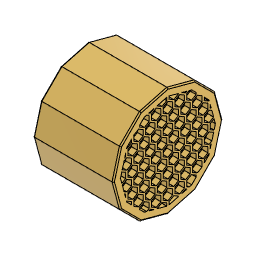
Speaker_End_Cap (Autodesk Fusion 360 design; units mm, degrees)
Autodesk Fusion 360 part; units mm, degrees
note: some values were not read from the file. Set by a fixed rule: which sketch regions a step uses.
sketch "Sketch1" plane through (0, 0, 0) normal (1, 0, 0) x (0, 1, 0)
  line L0 (22, 0) -> (19.0526, 11)
  line L1 (19.0526, 11) -> (11, 19.0526)
  line L2 (11, 19.0526) -> (0, 22)
  line L3 (0, 22) -> (-11, 19.0526)
  line L4 (-11, 19.0526) -> (-19.0526, 11)
  line L5 (-19.0526, 11) -> (-22, 0)
  line L6 (-22, 0) -> (-19.0526, -11)
  line L7 (-19.0526, -11) -> (-11, -19.0526)
  line L8 (-11, -19.0526) -> (0, -22)
  line L9 (0, -22) -> (11, -19.0526)
  line L10 (11, -19.0526) -> (19.0526, -11)
  line L11 (19.0526, -11) -> (22, 0)
  line L12 (20.1733, 11.647) -> (11.647, 20.1733)
  line L13 (11.647, 20.1733) -> (0, 23.2941)
  line L14 (0, 23.2941) -> (-11.647, 20.1733)
  line L15 (-11.647, 20.1733) -> (-20.1733, 11.647)
  line L16 (-20.1733, 11.647) -> (-23.2941, 0)
  line L17 (-23.2941, 0) -> (-20.1733, -11.647)
  line L18 (-20.1733, -11.647) -> (-11.647, -20.1733)
  line L19 (-11.647, -20.1733) -> (0, -23.2941)
  line L20 (0, -23.2941) -> (11.647, -20.1733)
  line L21 (11.647, -20.1733) -> (20.1733, -11.647)
  line L22 (20.1733, -11.647) -> (23.2941, 0)
  line L23 (23.2941, 0) -> (20.1733, 11.647)
  dimension "d1" = 22
  dimension "d2" = 1.25
  measures "d1" distance of L0.start origin
extrude "Extrude1" add sketch "Sketch1" along normal blind 2.5 contours L0 L1 L2 L3 L4 L5 L6 L7 L8 L9 L10 L11 | L12 L13 L14 L15 L16 L17 L18 L19 L20 L21 L22 L23
extrude "Extrude3" add sketch "Sketch1" against normal blind 31.5
fillet "Rounded Edges" radius 0.5 12 edges at (2.5, -5.8235, 21.7337) (2.5, 5.8235, 21.7337) (2.5, 15.9102, 15.9102) (2.5, 21.7337, 5.8235) (2.5, 21.7337, -5.8235) (2.5, 15.9102, -15.9102) (2.5, 5.8235, -21.7337) (2.5, -5.8235, -21.7337) (2.5, -15.9102, -15.9102) (2.5, -21.7337, -5.8235) (2.5, -21.7337, 5.8235) (2.5, -15.9102, 15.9102)
fillet "Rounded Edges" radius 0.5 12 edges at (-31.5, -15.9102, 15.9102) (-31.5, -5.8235, 21.7337) (-31.5, 5.8235, 21.7337) (-31.5, 15.9102, 15.9102) (-31.5, 21.7337, 5.8235) (-31.5, 21.7337, -5.8235) (-31.5, 15.9102, -15.9102) (-31.5, 5.8235, -21.7337) (-31.5, -5.8235, -21.7337) (-31.5, -15.9102, -15.9102) (-31.5, -21.7337, -5.8235) (-31.5, -21.7337, 5.8235)
sketch "Speaker Grill" plane through (2.5, 0, 0) normal (1, 0, 0) x (0, 1, 0)
  line L0 (0, -22.7765) -> (11.3882, -19.725)
  line L1 (11.3882, -19.725) -> (19.725, -11.3882)
  line L2 (19.725, -11.3882) -> (22.7765, 0)
  line L3 (22.7765, 0) -> (19.725, 11.3882)
  line L4 (19.725, 11.3882) -> (11.3882, 19.725)
  line L5 (11.3882, 19.725) -> (0, 22.7765)
  line L6 (0, 22.7765) -> (-11.3882, 19.725)
  line L7 (-11.3882, 19.725) -> (-19.725, 11.3882)
  line L8 (-19.725, 11.3882) -> (-22.7765, 0)
  line L9 (-22.7765, 0) -> (-19.725, -11.3882)
  line L10 (-19.725, -11.3882) -> (-11.3882, -19.725)
  line L11 (-11.3882, -19.725) -> (0, -22.7765)
  line L12 (-17.4836, 10.0941) -> (-20.1883, 0)
  line L13 (-20.1883, 0) -> (-17.4836, -10.0941)
  line L14 (-17.4836, -10.0941) -> (-10.0941, -17.4836)
  line L15 (-10.0941, -17.4836) -> (0, -20.1883)
  line L16 (0, -20.1883) -> (10.0941, -17.4836)
  line L17 (10.0941, -17.4836) -> (17.4836, -10.0941)
  line L18 (17.4836, -10.0941) -> (20.1883, 0)
  line L19 (20.1883, 0) -> (17.4836, 10.0941)
  line L20 (17.4836, 10.0941) -> (10.0941, 17.4836)
  line L21 (10.0941, 17.4836) -> (0, 20.1883)
  line L22 (0, 20.1883) -> (-10.0941, 17.4836)
  line L23 (-10.0941, 17.4836) -> (-17.4836, 10.0941)
  line L24 (2, 1.1547) -> (0, 2.3094)
  line L25 (0, 2.3094) -> (-2, 1.1547)
  line L26 (-2, 1.1547) -> (-2, -1.1547)
  line L27 (-2, -1.1547) -> (0, -2.3094)
  line L28 (0, -2.3094) -> (2, -1.1547)
  line L29 (2, -1.1547) -> (2, 1.1547)
  line L30 (7, 1.1547) -> (5, 2.3094)
  line L31 (5, 2.3094) -> (3, 1.1547)
  line L32 (3, 1.1547) -> (3, -1.1547)
  line L33 (3, -1.1547) -> (5, -2.3094)
  line L34 (5, -2.3094) -> (7, -1.1547)
  line L35 (7, -1.1547) -> (7, 1.1547)
  line L36 (12, 1.1547) -> (10, 2.3094)
  line L37 (10, 2.3094) -> (8, 1.1547)
  line L38 (8, 1.1547) -> (8, -1.1547)
  line L39 (8, -1.1547) -> (10, -2.3094)
  line L40 (10, -2.3094) -> (12, -1.1547)
  line L41 (12, -1.1547) -> (12, 1.1547)
  line L42 (17, 1.1547) -> (15, 2.3094)
  line L43 (15, 2.3094) -> (13, 1.1547)
  line L44 (13, 1.1547) -> (13, -1.1547)
  line L45 (13, -1.1547) -> (15, -2.3094)
  line L46 (15, -2.3094) -> (17, -1.1547)
  line L47 (17, -1.1547) -> (17, 1.1547)
  line L48 (-7, -1.1547) -> (-5, -2.3094)
  line L49 (-5, -2.3094) -> (-3, -1.1547)
  line L50 (-3, -1.1547) -> (-3, 1.1547)
  line L51 (-3, 1.1547) -> (-5, 2.3094)
  line L52 (-5, 2.3094) -> (-7, 1.1547)
  line L53 (-7, 1.1547) -> (-7, -1.1547)
  line L54 (-12, -1.1547) -> (-10, -2.3094)
  line L55 (-10, -2.3094) -> (-8, -1.1547)
  line L56 (-8, -1.1547) -> (-8, 1.1547)
  line L57 (-8, 1.1547) -> (-10, 2.3094)
  line L58 (-10, 2.3094) -> (-12, 1.1547)
  line L59 (-12, 1.1547) -> (-12, -1.1547)
  line L60 (-17, -1.1547) -> (-15, -2.3094)
  line L61 (-15, -2.3094) -> (-13, -1.1547)
  line L62 (-13, -1.1547) -> (-13, 1.1547)
  line L63 (-13, 1.1547) -> (-15, 2.3094)
  line L64 (-15, 2.3094) -> (-17, 1.1547)
  line L65 (-17, 1.1547) -> (-17, -1.1547)
  line L66 (-18, 1.1547) -> (-20, 2.3094)
  line L67 (-20, 2.3094) -> (-22, 1.1547)
  line L68 (-22, 1.1547) -> (-22, -1.1547)
  line L69 (-22, -1.1547) -> (-20, -2.3094)
  line L70 (-20, -2.3094) -> (-18, -1.1547)
  line L71 (-18, -1.1547) -> (-18, 1.1547)
  line L72 (18, -1.1547) -> (20, -2.3094)
  line L73 (20, -2.3094) -> (22, -1.1547)
  line L74 (22, -1.1547) -> (22, 1.1547)
  line L75 (22, 1.1547) -> (20, 2.3094)
  line L76 (20, 2.3094) -> (18, 1.1547)
  line L77 (18, 1.1547) -> (18, -1.1547)
  line L78 (2.493, -1.6981) -> (0.4965, -2.8589)
  line L79 (0.4965, -2.8589) -> (0.5035, -5.1683)
  line L80 (0.5035, -5.1683) -> (2.507, -6.3169)
  line L81 (2.507, -6.3169) -> (4.5035, -5.1561)
  line L82 (4.5035, -5.1561) -> (4.4965, -2.8467)
  line L83 (4.4965, -2.8467) -> (2.493, -1.6981)
  line L84 (9.5035, -5.1561) -> (9.4965, -2.8467)
  line L85 (7.507, -6.3169) -> (9.5035, -5.1561)
  line L86 (5.5035, -5.1683) -> (7.507, -6.3169)
  line L87 (5.4965, -2.8589) -> (5.5035, -5.1683)
  line L88 (7.493, -1.6981) -> (5.4965, -2.8589)
  line L89 (9.4965, -2.8467) -> (7.493, -1.6981)
  line L90 (10.4965, -2.8589) -> (10.5035, -5.1683)
  line L91 (14.4965, -2.8467) -> (12.493, -1.6981)
  line L92 (12.507, -6.3169) -> (14.5035, -5.1561)
  line L93 (10.5035, -5.1683) -> (12.507, -6.3169)
  line L94 (12.493, -1.6981) -> (10.4965, -2.8589)
  line L95 (14.5035, -5.1561) -> (14.4965, -2.8467)
  line L96 (9.5, 2.8453) -> (9.5, 5.1547)
  line L97 (-4.5, 5.1547) -> (-4.5, 2.8453)
  line L98 (-2.5, 6.3094) -> (-4.5, 5.1547)
  line L99 (-2.5, 1.6906) -> (-0.5, 2.8453)
  line L100 (-5.5, 5.1547) -> (-7.5, 6.3094)
  line L101 (-9.5, 2.8453) -> (-7.5, 1.6906)
  line L102 (-7.5, 6.3094) -> (-9.5, 5.1547)
  line L103 (-7.5, 1.6906) -> (-5.5, 2.8453)
  line L104 (-4.5, 2.8453) -> (-2.5, 1.6906)
  line L105 (-0.5, 2.8453) -> (-0.5, 5.1547)
  line L106 (5.5, 5.1547) -> (5.5, 2.8453)
  line L107 (4.5, 2.8453) -> (4.5, 5.1547)
  line L108 (-9.5, 5.1547) -> (-9.5, 2.8453)
  line L109 (-5.5, 2.8453) -> (-5.5, 5.1547)
  line L110 (0.5, 5.1547) -> (0.5, 2.8453)
  line L111 (9.5, 5.1547) -> (7.5, 6.3094)
  line L112 (2.5, 1.6906) -> (4.5, 2.8453)
  line L113 (5.5, 2.8453) -> (7.5, 1.6906)
  line L114 (0.5, 2.8453) -> (2.5, 1.6906)
  line L115 (4.5, 5.1547) -> (2.5, 6.3094)
  line L116 (7.5, 6.3094) -> (5.5, 5.1547)
  line L117 (2.5, 6.3094) -> (0.5, 5.1547)
  line L118 (7.5, 1.6906) -> (9.5, 2.8453)
  line L119 (-0.5, 5.1547) -> (-2.5, 6.3094)
  line L120 (10.5, 2.8453) -> (12.5, 1.6906)
  line L121 (10.5, 5.1547) -> (10.5, 2.8453)
  line L122 (12.5, 6.3094) -> (10.5, 5.1547)
  line L123 (14.5, 5.1547) -> (12.5, 6.3094)
  line L124 (14.5, 2.8453) -> (14.5, 5.1547)
  line L125 (12.5, 1.6906) -> (14.5, 2.8453)
  line L126 (-10.5, 5.1547) -> (-12.5, 6.3094)
  line L127 (-12.5, 6.3094) -> (-14.5, 5.1547)
  line L128 (-14.5, 5.1547) -> (-14.5, 2.8453)
  line L129 (-14.5, 2.8453) -> (-12.5, 1.6906)
  line L130 (-12.5, 1.6906) -> (-10.5, 2.8453)
  line L131 (-10.5, 2.8453) -> (-10.5, 5.1547)
  line L132 (-15.5, 5.1547) -> (-17.5, 6.3094)
  line L133 (-17.5, 6.3094) -> (-19.5, 5.1547)
  line L134 (-19.5, 5.1547) -> (-19.5, 2.8453)
  line L135 (-19.5, 2.8453) -> (-17.5, 1.6906)
  line L136 (-17.5, 1.6906) -> (-15.5, 2.8453)
  line L137 (-15.5, 2.8453) -> (-15.5, 5.1547)
  line L138 (19.5, 2.8453) -> (19.5, 5.1547)
  line L139 (19.5, 5.1547) -> (17.5, 6.3094)
  line L140 (17.5, 6.3094) -> (15.5, 5.1547)
  line L141 (15.5, 5.1547) -> (15.5, 2.8453)
  line L142 (15.5, 2.8453) -> (17.5, 1.6906)
  line L143 (17.5, 1.6906) -> (19.5, 2.8453)
  line L144 (19.5035, -5.1561) -> (19.4965, -2.8467)
  line L145 (19.4965, -2.8467) -> (17.493, -1.6981)
  line L146 (17.493, -1.6981) -> (15.4965, -2.8589)
  line L147 (15.4965, -2.8589) -> (15.5035, -5.1683)
  line L148 (15.5035, -5.1683) -> (17.507, -6.3169)
  line L149 (17.507, -6.3169) -> (19.5035, -5.1561)
  line L150 (-15.4965, -5.1561) -> (-15.5035, -2.8467)
  line L151 (-15.5035, -2.8467) -> (-17.507, -1.6981)
  line L152 (-17.507, -1.6981) -> (-19.5035, -2.8589)
  line L153 (-19.5035, -2.8589) -> (-19.4965, -5.1683)
  line L154 (-19.4965, -5.1683) -> (-17.493, -6.3169)
  line L155 (-17.493, -6.3169) -> (-15.4965, -5.1561)
  line L156 (-14.5035, -2.8589) -> (-14.4965, -5.1683)
  line L157 (-12.507, -1.6981) -> (-14.5035, -2.8589)
  line L158 (-10.5035, -2.8467) -> (-12.507, -1.6981)
  line L159 (-10.4965, -5.1561) -> (-10.5035, -2.8467)
  line L160 (-12.493, -6.3169) -> (-10.4965, -5.1561)
  line L161 (-14.4965, -5.1683) -> (-12.493, -6.3169)
  line L162 (-9.4965, -5.1683) -> (-7.493, -6.3169)
  line L163 (-9.5035, -2.8589) -> (-9.4965, -5.1683)
  line L164 (-7.507, -1.6981) -> (-9.5035, -2.8589)
  line L165 (-5.5035, -2.8467) -> (-7.507, -1.6981)
  line L166 (-5.4965, -5.1561) -> (-5.5038, -2.7646)
  line L167 (-7.493, -6.3169) -> (-5.4965, -5.1561)
  line L168 (-4.5035, -2.8589) -> (-4.4965, -5.1683)
  line L169 (-2.507, -1.6981) -> (-4.5035, -2.8589)
  line L170 (-0.5035, -2.8467) -> (-2.507, -1.6981)
  line L171 (-0.4965, -5.1561) -> (-0.5035, -2.8467)
  line L172 (-2.493, -6.3169) -> (-0.4965, -5.1561)
  line L173 (-4.4965, -5.1683) -> (-2.493, -6.3169)
  line L174 (-4.5, 13.1547) -> (-4.5, 10.8453)
  line L175 (-2.5, 14.3094) -> (-4.5, 13.1547)
  line L176 (9.5, 10.8453) -> (9.5, 13.1547)
  line L177 (10.5, 13.1547) -> (10.5, 10.8453)
  line L178 (-2.5, 9.6906) -> (-0.5, 10.8453)
  line L179 (-15.5, 10.8453) -> (-15.5, 13.1547)
  line L180 (-5.007, 10.3019) -> (-7.0035, 9.1411)
  line L181 (2.5, 9.6906) -> (4.5, 10.8453)
  line L182 (-3.0035, 9.1533) -> (-5.007, 10.3019)
  line L183 (8, 14.8453) -> (10, 13.6906)
  line L184 (-6.9965, 6.8317) -> (-4.993, 5.6831)
  line L185 (3, 14.8453) -> (5, 13.6906)
  line L186 (-12.5, 14.3094) -> (-14.5, 13.1547)
  line L187 (-2, 17.1547) -> (-2, 14.8453)
  line L188 (2, 17.1547) -> (0, 18.3094)
  line L189 (7.5, 9.6906) -> (9.5, 10.8453)
  line L190 (-0.007, 10.3019) -> (-2.0035, 9.1411)
  line L191 (-8.0035, 9.1533) -> (-10.007, 10.3019)
  line L192 (-7.0035, 9.1411) -> (-6.9965, 6.8317)
  line L193 (-14.5, 10.8453) -> (-12.5, 9.6906)
  line L194 (-7, 17.1547) -> (-7, 14.8453)
  line L195 (0.007, 5.6831) -> (2.0035, 6.8439)
  line L196 (0.5, 10.8453) -> (2.5, 9.6906)
  line L197 (4.5, 13.1547) -> (2.5, 14.3094)
  line L198 (7.5, 14.3094) -> (5.5, 13.1547)
  line L199 (-14.993, 5.6831) -> (-12.9965, 6.8439)
  line L200 (7, 17.1547) -> (5, 18.3094)
  line L201 (2, 14.8453) -> (2, 17.1547)
  line L202 (-12.5, 9.6906) -> (-10.5, 10.8453)
  line L203 (-17.0035, 9.1411) -> (-16.9965, 6.8317)
  line L204 (-12.9965, 6.8439) -> (-13.0035, 9.1533)
  line L205 (0, 13.6906) -> (2, 14.8453)
  line L206 (6.9965, 9.1533) -> (4.993, 10.3019)
  line L207 (-1.9965, 6.8317) -> (0.007, 5.6831)
  line L208 (4.993, 10.3019) -> (2.9965, 9.1411)
  line L209 (-10, 13.6906) -> (-8, 14.8453)
  line L210 (-10, 18.3094) -> (-12, 17.1547)
  line L211 (8.0035, 6.8317) -> (10.007, 5.6831)
  line L212 (5, 13.6906) -> (7, 14.8453)
  line L213 (-7.5, 9.6906) -> (-5.5, 10.8453)
  line L214 (-10.5, 13.1547) -> (-12.5, 14.3094)
  line L215 (-7.9965, 6.8439) -> (-8.0035, 9.1533)
  line L216 (-16.9965, 6.8317) -> (-14.993, 5.6831)
  line L217 (5.007, 5.6831) -> (7.0035, 6.8439)
  line L218 (5, 18.3094) -> (3, 17.1547)
  line L219 (-5, 13.6906) -> (-3, 14.8453)
  line L220 (-12.0035, 9.1411) -> (-11.9965, 6.8317)
  line L221 (-3, 17.1547) -> (-5, 18.3094)
  line L222 (-12, 17.1547) -> (-12, 14.8453)
  line L223 (-9.993, 5.6831) -> (-7.9965, 6.8439)
  line L224 (7, 14.8453) -> (7, 17.1547)
  line L225 (-5.5, 13.1547) -> (-7.5, 14.3094)
  line L226 (-3, 14.8453) -> (-3, 17.1547)
  line L227 (10, 18.3094) -> (8, 17.1547)
  line L228 (-15.007, 10.3019) -> (-17.0035, 9.1411)
  line L229 (-2.9965, 6.8439) -> (-3.0035, 9.1533)
  line L230 (7.0035, 6.8439) -> (6.9965, 9.1533)
  line L231 (1.9965, 9.1533) -> (-0.007, 10.3019)
  line L232 (9.993, 10.3019) -> (7.9965, 9.1411)
  line L233 (-11.9965, 6.8317) -> (-9.993, 5.6831)
  line L234 (-13.0035, 9.1533) -> (-15.007, 10.3019)
  line L235 (5.5, 10.8453) -> (7.5, 9.6906)
  line L236 (-4.993, 5.6831) -> (-2.9965, 6.8439)
  line L237 (-5, 18.3094) -> (-7, 17.1547)
  line L238 (-10.007, 10.3019) -> (-12.0035, 9.1411)
  line L239 (9.5, 13.1547) -> (7.5, 14.3094)
  line L240 (5.5, 13.1547) -> (5.5, 10.8453)
  line L241 (-7, 14.8453) -> (-5, 13.6906)
  line L242 (-2, 14.8453) -> (0, 13.6906)
  line L243 (4.5, 10.8453) -> (4.5, 13.1547)
  line L244 (-0.5, 10.8453) -> (-0.5, 13.1547)
  line L245 (0.5, 13.1547) -> (0.5, 10.8453)
  line L246 (-14.5, 13.1547) -> (-14.5, 10.8453)
  line L247 (-9.5, 13.1547) -> (-9.5, 10.8453)
  line L248 (-10.5, 10.8453) -> (-10.5, 13.1547)
  line L249 (-5.5, 10.8453) -> (-5.5, 13.1547)
  line L250 (-8, 14.8453) -> (-8, 17.1547)
  line L251 (-15.5, 13.1547) -> (-17.5, 14.3094)
  line L252 (-8, 17.1547) -> (-10, 18.3094)
  line L253 (-7.5, 14.3094) -> (-9.5, 13.1547)
  line L254 (-9.5, 10.8453) -> (-7.5, 9.6906)
  line L255 (2.5, 14.3094) -> (0.5, 13.1547)
  line L256 (3.0035, 6.8317) -> (5.007, 5.6831)
  line L257 (2.9965, 9.1411) -> (3.0035, 6.8317)
  line L258 (0, 18.3094) -> (-2, 17.1547)
  line L259 (-4.5, 10.8453) -> (-2.5, 9.6906)
  line L260 (-17.5, 9.6906) -> (-15.5, 10.8453)
  line L261 (7.9965, 9.1411) -> (8.0035, 6.8317)
  line L262 (-2.0035, 9.1411) -> (-1.9965, 6.8317)
  line L263 (-0.5, 13.1547) -> (-2.5, 14.3094)
  line L264 (2.0035, 6.8439) -> (1.9965, 9.1533)
  line L265 (3, 17.1547) -> (3, 14.8453)
  line L266 (8, 17.1547) -> (8, 14.8453)
  line L267 (-12, 14.8453) -> (-10, 13.6906)
  line L268 (14.5, 10.8453) -> (14.5, 13.1547)
  line L269 (14.993, 10.3019) -> (12.9965, 9.1411)
  line L270 (19.5, 13.1547) -> (17.5, 14.3094)
  line L271 (12, 14.8453) -> (12, 17.1547)
  line L272 (16.9965, 9.1533) -> (14.993, 10.3019)
  line L273 (19.5, 10.8453) -> (19.5, 13.1547)
  line L274 (12.0035, 6.8439) -> (11.9965, 9.1533)
  line L275 (17.0035, 6.8439) -> (16.9965, 9.1533)
  line L276 (12.5, 9.6906) -> (14.5, 10.8453)
  line L277 (12.9965, 9.1411) -> (13.0035, 6.8317)
  line L278 (14.5, 13.1547) -> (12.5, 14.3094)
  line L279 (15.5, 10.8453) -> (17.5, 9.6906)
  line L280 (17.5, 14.3094) -> (15.5, 13.1547)
  line L281 (17.5, 9.6906) -> (19.5, 10.8453)
  line L282 (15.5, 13.1547) -> (15.5, 10.8453)
  line L283 (13.0035, 6.8317) -> (15.007, 5.6831)
  line L284 (15.007, 5.6831) -> (17.0035, 6.8439)
  line L285 (10.5, 10.8453) -> (12.5, 9.6906)
  line L286 (12.5, 14.3094) -> (10.5, 13.1547)
  line L287 (10, 13.6906) -> (12, 14.8453)
  line L288 (12, 17.1547) -> (10, 18.3094)
  line L289 (10.007, 5.6831) -> (12.0035, 6.8439)
  line L290 (11.9965, 9.1533) -> (9.993, 10.3019)
  line L291 (-17.9965, 6.8439) -> (-18.0035, 9.1533)
  line L292 (-18.0035, 9.1533) -> (-20.007, 10.3019)
  line L293 (-20.007, 10.3019) -> (-22.0035, 9.1411)
  line L294 (-22.0035, 9.1411) -> (-21.9965, 6.8317)
  line L295 (-21.9965, 6.8317) -> (-19.993, 5.6831)
  line L296 (-19.993, 5.6831) -> (-17.9965, 6.8439)
  line L297 (-19.5, 10.8453) -> (-17.5, 9.6906)
  line L298 (-19.5, 13.1547) -> (-19.5, 10.8453)
  line L299 (-17.5, 14.3094) -> (-19.5, 13.1547)
  line L300 (4.5, 21.1547) -> (2.5, 22.3094)
  line L301 (2.5, 22.3094) -> (0.5, 21.1547)
  line L302 (0.5, 21.1547) -> (0.5, 18.8453)
  line L303 (0.5, 18.8453) -> (2.5, 17.6906)
  line L304 (2.5, 17.6906) -> (4.5, 18.8453)
  line L305 (4.5, 18.8453) -> (4.5, 21.1547)
  line L306 (-0.5, 21.1547) -> (-2.5, 22.3094)
  line L307 (-2.5, 22.3094) -> (-4.5, 21.1547)
  line L308 (-4.5, 21.1547) -> (-4.5, 18.8453)
  line L309 (-4.5, 18.8453) -> (-2.5, 17.6906)
  line L310 (-2.5, 17.6906) -> (-0.5, 18.8453)
  line L311 (-0.5, 18.8453) -> (-0.5, 21.1547)
  line L312 (5.5, 21.1547) -> (5.5, 18.8453)
  line L313 (9.5, 21.1547) -> (7.5, 22.3094)
  line L314 (7.5, 22.3094) -> (5.5, 21.1547)
  line L315 (5.5, 18.8453) -> (7.5, 17.6906)
  line L316 (7.5, 17.6906) -> (9.5, 18.8453)
  line L317 (9.5, 18.8453) -> (9.5, 21.1547)
  line L318 (-5.5, 21.1547) -> (-7.5, 22.3094)
  line L319 (-7.5, 22.3094) -> (-9.5, 21.1547)
  line L320 (-9.5, 21.1547) -> (-9.5, 18.8453)
  line L321 (-9.5, 18.8453) -> (-7.5, 17.6906)
  line L322 (-7.5, 17.6906) -> (-5.5, 18.8453)
  line L323 (-5.5, 18.8453) -> (-5.5, 21.1547)
  line L324 (7.0035, -9.1561) -> (6.9965, -6.8467)
  line L325 (-5, -18.3094) -> (-3, -17.1547)
  line L326 (-19.5, -10.8453) -> (-19.5, -13.1547)
  line L327 (12.0035, -9.1561) -> (11.9965, -6.8467)
  line L328 (12, -17.1547) -> (12, -14.8453)
  line L329 (7, -17.1547) -> (7, -14.8453)
  line L330 (-4.4965, -21.1683) -> (-2.493, -22.3169)
  line L331 (-5, -13.6906) -> (-7, -14.8453)
  line L332 (12.9965, -6.8589) -> (13.0035, -9.1683)
  line L333 (7.507, -22.3169) -> (9.5035, -21.1561)
  line L334 (-9.5035, -18.8589) -> (-9.4965, -21.1683)
  line L335 (2, -17.1547) -> (2, -14.8453)
  line L336 (-7, -17.1547) -> (-5, -18.3094)
  line L337 (-12, -17.1547) -> (-10, -18.3094)
  line L338 (-5.5, -13.1547) -> (-5.5, -10.8453)
  line L339 (-9.5, -13.1547) -> (-7.5, -14.3094)
  line L340 (2.493, -17.6981) -> (0.4965, -18.8589)
  line L341 (3, -14.8453) -> (3, -17.1547)
  line L342 (-15.5, -13.1547) -> (-15.5, -10.8453)
  line L343 (2.0035, -9.1561) -> (1.9965, -6.8467)
  line L344 (-12.8895, -14.6882) -> (-12.8895, -14.6712)
  line L345 (-2.493, -22.3169) -> (-0.4965, -21.1561)
  line L346 (8, -14.8453) -> (8, -17.1547)
  line L347 (-9.5, -10.8453) -> (-9.5, -13.1547)
  line L348 (-4.5, -10.8453) -> (-4.5, -13.1547)
  line L349 (4.4965, -18.8467) -> (2.493, -17.6981)
  line L350 (-0.4965, -21.1561) -> (-0.5035, -18.8467)
  line L351 (-17.5, -14.3094) -> (-15.5, -13.1547)
  line L352 (-15.5, -10.8453) -> (-17.5, -9.6906)
  line L353 (10, -18.3094) -> (12, -17.1547)
  line L354 (9.5035, -21.1561) -> (9.4965, -18.8467)
  line L355 (7.493, -17.6981) -> (5.4965, -18.8589)
  line L356 (5.5035, -21.1683) -> (7.507, -22.3169)
  line L357 (5, -18.3094) -> (7, -17.1547)
  line L358 (0.4965, -18.8589) -> (0.5035, -21.1683)
  line L359 (8, -17.1547) -> (10, -18.3094)
  line L360 (2.507, -22.3169) -> (4.5035, -21.1561)
  line L361 (0, -18.3094) -> (2, -17.1547)
  line L362 (0, -13.6906) -> (-2, -14.8453)
  line L363 (5.4965, -18.8589) -> (5.5035, -21.1683)
  line L364 (1.9965, -6.8467) -> (-0.007, -5.6981)
  line L365 (-1.9965, -9.1683) -> (0.007, -10.3169)
  line L366 (9.4965, -18.8467) -> (7.493, -17.6981)
  line L367 (-12, -14.8453) -> (-12, -17.1547)
  line L368 (0.5035, -21.1683) -> (2.507, -22.3169)
  line L369 (-2, -14.8453) -> (-2, -17.1547)
  line L370 (3, -17.1547) -> (5, -18.3094)
  line L371 (12.8895, -14.6712) -> (12.8895, -14.6882)
  line L372 (-3, -17.1547) -> (-3, -14.8453)
  line L373 (-8, -17.1547) -> (-8, -14.8453)
  line L374 (-7.507, -17.6981) -> (-9.5035, -18.8589)
  line L375 (4.5035, -21.1561) -> (4.4965, -18.8467)
  line L376 (-7, -14.8453) -> (-7, -17.1547)
  line L377 (-21.9965, -9.1683) -> (-19.993, -10.3169)
  line L378 (-17.0035, -6.8589) -> (-16.9965, -9.1683)
  line L379 (-11.9965, -9.1683) -> (-9.993, -10.3169)
  line L380 (-2.9965, -9.1561) -> (-3.0035, -6.8467)
  line L381 (-0.007, -5.6981) -> (-2.0035, -6.8589)
  line L382 (-4.993, -10.3169) -> (-2.9965, -9.1561)
  line L383 (-7.0035, -6.8589) -> (-6.9965, -9.1683)
  line L384 (-17.9965, -9.1561) -> (-18.0035, -6.8467)
  line L385 (-7.9965, -9.1561) -> (-8.0035, -6.8467)
  line L386 (-19.993, -10.3169) -> (-17.9965, -9.1561)
  line L387 (-10.007, -5.6981) -> (-12.0035, -6.8589)
  line L388 (-18.0035, -6.8467) -> (-20.007, -5.6981)
  line L389 (-2.0035, -6.8589) -> (-1.9965, -9.1683)
  line L390 (-12.0035, -6.8589) -> (-11.9965, -9.1683)
  line L391 (-13.0035, -6.8467) -> (-15.007, -5.6981)
  line L392 (-8.0035, -6.8467) -> (-10.007, -5.6981)
  line L393 (-2.507, -17.6981) -> (-4.5035, -18.8589)
  line L394 (9.5, -10.8453) -> (7.5, -9.6906)
  line L395 (-14.993, -10.3169) -> (-12.9965, -9.1561)
  line L396 (-10.5, -10.8453) -> (-12.5, -9.6906)
  line L397 (-10, -13.6906) -> (-12, -14.8453)
  line L398 (15.5, -13.1547) -> (17.5, -14.3094)
  line L399 (7.5, -14.3094) -> (9.5, -13.1547)
  line L400 (19.5, -10.8453) -> (17.5, -9.6906)
  line L401 (9.5, -13.1547) -> (9.5, -10.8453)
  line L402 (10.5, -10.8453) -> (10.5, -13.1547)
  line L403 (10.5, -13.1547) -> (12.5, -14.3094)
  line L404 (10.007, -10.3169) -> (12.0035, -9.1561)
  line L405 (17.5, -9.6906) -> (15.5, -10.8453)
  line L406 (14.5, -10.8453) -> (12.5, -9.6906)
  line L407 (-4.5, -13.1547) -> (-2.5, -14.3094)
  line L408 (12.5, -9.6906) -> (10.5, -10.8453)
  line L409 (-3.0035, -6.8467) -> (-5.007, -5.6981)
  line L410 (15.5, -10.8453) -> (15.5, -13.1547)
  line L411 (0.5, -13.1547) -> (2.5, -14.3094)
  line L412 (10, -13.6906) -> (8, -14.8453)
  line L413 (14.5, -13.1547) -> (14.5, -10.8453)
  line L414 (-6.9965, -9.1683) -> (-4.993, -10.3169)
  line L415 (-2.5, -14.3094) -> (-0.5, -13.1547)
  line L416 (-12.5, -9.6906) -> (-14.5, -10.8453)
  line L417 (-9.993, -10.3169) -> (-7.9965, -9.1561)
  line L418 (-5.007, -5.6981) -> (-7.0035, -6.8589)
  line L419 (-10.5, -13.1547) -> (-10.5, -10.8453)
  line L420 (2.5, -14.3094) -> (4.5, -13.1547)
  line L421 (12.5, -14.3094) -> (14.5, -13.1547)
  line L422 (12.9296, -14.6481) -> (12.8895, -14.6712)
  line L423 (5.5, -10.8453) -> (5.5, -13.1547)
  line L424 (-7.5, -14.3094) -> (-5.5, -13.1547)
  line L425 (16.9965, -6.8467) -> (14.993, -5.6981)
  line L426 (17.5, -14.3094) -> (19.5, -13.1547)
  line L427 (-12.9965, -9.1561) -> (-13.0035, -6.8467)
  line L428 (11.9965, -6.8467) -> (9.993, -5.6981)
  line L429 (19.5, -13.1547) -> (19.5, -10.8453)
  line L430 (0.5, -10.8453) -> (0.5, -13.1547)
  line L431 (4.5, -10.8453) -> (2.5, -9.6906)
  line L432 (-22.0035, -6.8589) -> (-21.9965, -9.1683)
  line L433 (5, -13.6906) -> (3, -14.8453)
  line L434 (13.0035, -9.1683) -> (15.007, -10.3169)
  line L435 (-7.5, -9.6906) -> (-9.5, -10.8453)
  line L436 (-14.5, -10.8453) -> (-14.5, -13.1547)
  line L437 (-16.9965, -9.1683) -> (-14.993, -10.3169)
  line L438 (6.9965, -6.8467) -> (4.993, -5.6981)
  line L439 (12, -14.8453) -> (10, -13.6906)
  line L440 (-15.007, -5.6981) -> (-17.0035, -6.8589)
  line L441 (-2.5, -9.6906) -> (-4.5, -10.8453)
  line L442 (-5.5035, -18.8467) -> (-7.507, -17.6981)
  line L443 (-0.5, -13.1547) -> (-0.5, -10.8453)
  line L444 (-7.493, -22.3169) -> (-5.4965, -21.1561)
  line L445 (-14.5, -13.1547) -> (-12.5, -14.3094)
  line L446 (-5.4965, -21.1561) -> (-5.5035, -18.8467)
  line L447 (-17.5, -9.6906) -> (-19.5, -10.8453)
  line L448 (3.0035, -9.1683) -> (5.007, -10.3169)
  line L449 (2.5, -9.6906) -> (0.5, -10.8453)
  line L450 (-19.5, -13.1547) -> (-17.5, -14.3094)
  line L451 (-10, -18.3094) -> (-8, -17.1547)
  line L452 (9.993, -5.6981) -> (7.9965, -6.8589)
  line L453 (-8, -14.8453) -> (-10, -13.6906)
  line L454 (-0.5, -10.8453) -> (-2.5, -9.6906)
  line L455 (4.993, -5.6981) -> (2.9965, -6.8589)
  line L456 (5.5, -13.1547) -> (7.5, -14.3094)
  line L457 (7.9965, -6.8589) -> (8.0035, -9.1683)
  line L458 (-20.007, -5.6981) -> (-22.0035, -6.8589)
  line L459 (5.007, -10.3169) -> (7.0035, -9.1561)
  line L460 (17.0035, -9.1561) -> (16.9965, -6.8467)
  line L461 (-3, -14.8453) -> (-5, -13.6906)
  line L462 (-0.5035, -18.8467) -> (-2.507, -17.6981)
  line L463 (7.5, -9.6906) -> (5.5, -10.8453)
  line L464 (-4.5035, -18.8589) -> (-4.4965, -21.1683)
  line L465 (4.5, -13.1547) -> (4.5, -10.8453)
  line L466 (8.0035, -9.1683) -> (10.007, -10.3169)
  line L467 (-12.5, -14.3094) -> (-10.5, -13.1547)
  line L468 (-5.5, -10.8453) -> (-7.5, -9.6906)
  line L469 (-9.4965, -21.1683) -> (-7.493, -22.3169)
  line L470 (-2, -17.1547) -> (0, -18.3094)
  line L471 (-12.8895, -14.6712) -> (-12.9296, -14.6481)
  line L472 (2.9965, -6.8589) -> (3.0035, -9.1683)
  line L473 (14.993, -5.6981) -> (12.9965, -6.8589)
  line L474 (0.007, -10.3169) -> (2.0035, -9.1561)
  line L475 (15.007, -10.3169) -> (17.0035, -9.1561)
  line L476 (7, -14.8453) -> (5, -13.6906)
  line L477 (2, -14.8453) -> (0, -13.6906)
  line L478 (22.0035, -9.1561) -> (21.9965, -6.8467)
  line L479 (21.9965, -6.8467) -> (19.993, -5.6981)
  line L480 (19.993, -5.6981) -> (17.9965, -6.8589)
  line L481 (17.9965, -6.8589) -> (18.0035, -9.1683)
  line L482 (18.0035, -9.1683) -> (20.007, -10.3169)
  line L483 (20.007, -10.3169) -> (22.0035, -9.1561)
  line L484 (21.9965, 9.1533) -> (19.993, 10.3019)
  line L485 (19.993, 10.3019) -> (17.9965, 9.1411)
  line L486 (17.9965, 9.1411) -> (18.0035, 6.8317)
  line L487 (18.0035, 6.8317) -> (20.007, 5.6831)
  line L488 (20.007, 5.6831) -> (22.0035, 6.8439)
  line L489 (22.0035, 6.8439) -> (21.9965, 9.1533)
  point P0 (5, 0)
  point P1 (10, 0)
  point P2 (15, 0)
  point P3 (-5, 0)
  point P4 (-10, 0)
  point P5 (-15, 0)
  point P6 (-20, 0)
  point P7 (20, 0)
  point P8 (2.5, -4.0075)
  point P9 (10, -2.3094)
  point P10 (9.5035, -5.1561)
  point P11 (9.4965, -2.8467)
  point P12 (2.5, 4)
  point P13 (-2.5, 4)
  point P14 (2.0035, -1.1561)
  point P15 (1.9965, 1.1533)
  point P16 (-0.007, 2.3019)
  point P17 (0.007, -2.3169)
  point P18 (0, -0.0075)
  point P19 (-2.0035, 1.1411)
  point P20 (-1.9965, -1.1683)
  point P21 (-2.5, 4)
  point P22 (7.5, 4)
  point P23 (6.9965, 1.1533)
  point P24 (7.9965, 1.1411)
  point P25 (7.5, 1.6906)
  point P26 (7.0035, -1.1561)
  point P27 (-7.5, 4)
  point P28 (2.9965, 1.1411)
  point P29 (3.0035, -1.1683)
  point P30 (4.993, 2.3019)
  point P31 (7.0035, -1.1561)
  point P32 (6.9965, 1.1533)
  point P33 (5.007, -2.3169)
  point P34 (11.9965, 1.1533)
  point P35 (10.007, -2.3169)
  point P36 (8.0035, -1.1683)
  point P37 (12.0035, -1.1561)
  point P38 (9.993, 2.3019)
  point P39 (17.9383, 12)
  point P40 (2.5, 12)
  point P41 (-2.5, 12)
  point P42 (-12.5, 12)
  point P43 (0, 7.9925)
  point P44 (-17.5, 12)
  point P45 (-2.5, 12)
  point P46 (7.5, 12)
  point P47 (17.5, 12)
  point P48 (0.4965, 13.1411)
  point P49 (2.493, 14.3019)
  point P50 (0.5035, 10.8317)
  point P51 (6.9965, 9.1533)
  point P52 (7.5, 9.6906)
  point P53 (7.0035, 6.8439)
  point P54 (4.4965, 13.1533)
  point P55 (5, 13.6906)
  point P56 (5.4965, 13.1411)
  point P57 (4.5035, 10.8439)
  point P58 (-10, 16)
  point P59 (-7.5, 12)
  point P60 (12.5, 12)
  point P61 (0, 16)
  point P62 (-5, 16)
  point P63 (-0.5035, 13.1533)
  point P64 (-2.493, 9.6831)
  point P65 (5, 16)
  point P66 (-4.5035, 13.1411)
  point P67 (-2.5, 11.9925)
  point P68 (-0.4965, 10.8439)
  point P69 (-4.4965, 10.8317)
  point P70 (-2.507, 14.3019)
  point P71 (-5, 16)
  point P72 (7.507, 9.6831)
  point P73 (9.5035, 10.8439)
  point P74 (7.493, 14.3019)
  point P75 (4.5035, 10.8439)
  point P76 (2.507, 9.6831)
  point P77 (5.5035, 10.8317)
  point P78 (9.4965, 13.1533)
  point P79 (4.4965, 13.1533)
  point P80 (-20.4383, -16)
  point P81 (-17.7001, -5.7809)
  point P82 (17.7001, -5.7809)
  point P83 (20.4383, -16)
  point P84 (5, -16)
  point P85 (2.5, -6.3094)
  point P86 (0, -16)
  point P87 (-10, -16)
  point P88 (2.5, -20.0075)
  point P89 (-15, -16)
  point P90 (0, -16)
  point P91 (10, -16)
  point P92 (20, -16)
  point P93 (12.5, -6.3094)
  point P94 (2.9965, -14.8589)
  point P95 (4.993, -13.6981)
  point P96 (3.0035, -17.1683)
  point P97 (9.4965, -18.8467)
  point P98 (10, -18.3094)
  point P99 (9.5035, -21.1561)
  point P100 (6.9965, -14.8467)
  point P101 (7.5, -14.3094)
  point P102 (7.9965, -14.8589)
  point P103 (7.0035, -17.1561)
  point P104 (-7.5, -12)
  point P105 (7.507, -6.3169)
  point P106 (2.507, -6.3169)
  point P107 (-5, -16)
  point P108 (-2.493, -6.3169)
  point P109 (15, -16)
  point P110 (-12.5, -6.3094)
  point P111 (-17.5, -6.3094)
  point P112 (-2.5, -6.3094)
  point P113 (2.5, -12)
  point P114 (-2.5, -12)
  point P115 (1.9965, -14.8467)
  point P116 (0.007, -18.3169)
  point P117 (7.5, -12)
  point P118 (-2.0035, -14.8589)
  point P119 (0, -16.0075)
  point P120 (2.0035, -17.1561)
  point P121 (-1.9965, -17.1683)
  point P122 (-0.007, -13.6981)
  point P123 (-2.5, -12)
  point P124 (6.9965, -6.8467)
  point P125 (7.5, -6.3094)
  point P126 (7.0035, -9.1561)
  point P127 (-7.5, -6.3094)
  point P128 (0, -8.0075)
  point P129 (7.5, -6.3094)
  point P130 (17.5, -6.3094)
  point P131 (10.007, -18.3169)
  point P132 (12.0035, -17.1561)
  point P133 (9.993, -13.6981)
  point P134 (7.0035, -17.1561)
  point P135 (5.007, -18.3169)
  point P136 (8.0035, -17.1683)
  point P137 (11.9965, -14.8467)
  point P138 (6.9965, -14.8467)
  point P139 (-20, -16)
  dimension "d13" = -2.5
  dimension "d15" = 2
  dimension "d16" = 2.5
  dimension "d20" = 2.5
  dimension "d21" = 2
  dimension "d22" = 2.5
  dimension "d23" = 2.5
  dimension "d24" = 2
  dimension "d25" = 2.5
  dimension "d26" = 2.5
  dimension "d27" = 2
  constraint coincident L14 L344.start
  constraint coincident L14 L471.end
  constraint coincident L17 L422.start
  constraint coincident L17 L371.end
  constraint coincident L165.start L166
  measures "d15" distance of P8 L83
  measures "d16" horizontal distance of origin P8
  measures "d20" horizontal distance of P18 P21
  measures "d21" distance of P43 L231
  measures "d22" horizontal distance of P43 P45
  measures "d23" horizontal distance of P67 P71
  measures "d24" distance of P88 L349
  measures "d25" horizontal distance of P88 P90
  measures "d26" horizontal distance of P119 P123
  measures "d27" distance of P128 L364
extrude "Speaker Grill Cutouts" cut sketch "Speaker Grill" against normal blind 6 contours L16 L340 L349 L358 L375 | L15 L350 L393 L462 L464 | L16 L355 L366 | L15 L374 L442 | L16 L17 L328 L346 L359 L412 L439 | L14 L15 L367 L373 L397 L451 L453 | L17 L18 L400 L405 L410 | L13 L14 L342 L352 L447 | L17 L413 L421 | L17 L402 L403 L406 L408 L413 L421 | L14 L396 L416 L419 L436 L445 L467 | L14 L436 L445 | L18 L480 L481 | L13 L384 L388 | L18 L145 L146 L147 L148 L149 | L13 L150 L151 L152 L154 L155 | L19 L486 L487 | L18 L19 L72 L76 L77 | L12 L291 L296 | L12 L13 L66 L70 L71 | L19 L139 L140 L141 L142 L143 | L12 L132 L133 L135 L136 L137 | L19 L20 L279 L281 L282 | L12 L23 L179 L260 L297 | L20 L177 L268 L276 L278 L285 L286 | L20 L268 L278 | L23 L186 L246 | L23 L186 L193 L202 L214 L246 L248 | L21 L315 L316 | L22 L321 L322 | L20 L21 L183 L227 L266 L271 L287 | L22 L23 L209 L222 L250 L252 L267 | L21 L302 L303 L304 L305 | L22 L308 L309 L310 L311 | L24 L25 L26 L27 L28 L29 | L30 L31 L32 L33 L34 L35 | L36 L37 L38 L39 L40 L41 | L42 L43 L44 L45 L46 L47 | L48 L49 L50 L51 L52 L53 | L54 L55 L56 L57 L58 L59 | L60 L61 L62 L63 L64 L65 | L78 L79 L80 L81 L82 L83 | L84 L85 L86 L87 L88 L89 | L90 L91 L92 L93 L94 L95 | L96 L106 L111 L113 L116 L118 | L97 L98 L99 L104 L105 L119 | L100 L101 L102 L103 L108 L109 | L107 L110 L112 L114 L115 L117 | L120 L121 L122 L123 L124 L125 | L126 L127 L128 L129 L130 L131 | L156 L157 L158 L159 L160 L161 | L162 L163 L164 L165 L166 L167 | L168 L169 L170 L171 L172 L173 | L174 L175 L178 L244 L259 L263 | L176 L189 L198 L235 L239 L240 | L180 L182 L184 L192 L229 L236 | L181 L196 L197 L243 L245 L255 | L185 L200 L212 L218 L224 L265 | L187 L188 L201 L205 L242 L258 | L190 L195 L207 L231 L262 L264 | L191 L215 L220 L223 L233 L238 | L194 L219 L221 L226 L237 L241 | L199 L203 L204 L216 L228 L234 | L206 L208 L217 L230 L256 L257 | L211 L232 L261 L274 L289 L290 | L213 L225 L247 L249 L253 L254 | L269 L272 L275 L277 L283 L284 | L324 L438 L448 L455 L459 L472 | L325 L331 L336 L372 L376 L461 | L327 L404 L428 L452 L457 L466 | L329 L341 L357 L370 L433 L476 | L332 L425 L434 L460 L473 L475 | L335 L361 L362 L369 L470 L477 | L338 L339 L347 L424 L435 L468 | L343 L364 L365 L381 L389 L474 | L348 L407 L415 L441 L443 L454 | L378 L391 L395 L427 L437 L440 | L379 L385 L387 L390 L392 L417 | L380 L382 L383 L409 L414 L418 | L394 L399 L401 L423 L456 L463 | L411 L420 L430 L431 L449 L465
named bodies: "Speaker End Cap"
